Autodesk Inventor part; units mm, degrees
(part 3 of 3)
  arc A521 (160.6305, 133.2562) -> (159.9026, 133.5577) centre (148.5, 105) ccw projected
  arc A522 (159.9026, 133.5577) -> (159.9766, 134.127) centre (152.4268, 134.8199) ccw projected
  arc A523 (159.9766, 134.127) -> (160.0175, 134.9083) centre (150.1116, 135.0348) ccw projected
  arc A524 (160.0175, 134.9083) -> (159.988, 135.9358) centre (147.6733, 135.0675) ccw projected
  arc A525 (159.988, 135.9358) -> (159.2452, 136.2016) centre (148.5, 105) ccw projected
  arc A526 (159.2452, 136.2016) -> (158.5704, 135.426) centre (168.2137, 127.718) ccw projected
  arc A527 (158.5704, 135.426) -> (158.1064, 134.7962) centre (166.3081, 129.2396) ccw projected
  arc A528 (158.1064, 134.7962) -> (157.8025, 134.3091) centre (164.3821, 130.5422) ccw projected
  arc A529 (157.8025, 134.3091) -> (157.0485, 134.5379) centre (148.5, 105) ccw projected
  arc A530 (157.0485, 134.5379) -> (157.0664, 135.1116) centre (149.485, 135.0612) ccw projected
  arc A531 (157.0664, 135.1116) -> (157.0305, 135.8932) centre (147.1599, 135.0481) ccw projected
  arc A532 (157.0305, 135.8932) -> (156.9004, 136.9129) centre (144.7301, 134.8417) ccw projected
  arc A533 (156.9004, 136.9129) -> (156.1351, 137.1046) centre (148.5, 105) ccw projected
  arc A534 (156.1351, 137.1046) -> (155.5397, 136.2666) centre (165.892, 129.5409) ccw projected
  arc A535 (155.5397, 136.2666) -> (155.1396, 135.5943) centre (163.8464, 130.8684) ccw projected
  arc A536 (155.1396, 135.5943) -> (154.8849, 135.0798) centre (161.802, 131.976) ccw projected
  arc A537 (154.8849, 135.0798) -> (154.1121, 135.2335) centre (148.5, 105) ccw projected
  arc A538 (154.1121, 135.2335) -> (154.0737, 135.8063) centre (146.5338, 135.013) ccw projected
  arc A539 (154.0737, 135.8063) -> (153.9614, 136.5805) centre (144.2211, 134.7721) ccw projected
  arc A540 (153.9614, 136.5805) -> (153.7319, 137.5826) centre (141.8233, 134.3285) ccw projected
  arc A541 (153.7319, 137.5826) -> (152.9516, 137.6984) centre (148.5, 105) ccw projected
  arc A542 (152.9516, 137.6984) -> (152.4411, 136.8061) centre (163.4028, 131.1274) ccw projected
  arc A543 (152.4411, 136.8061) -> (152.1089, 136.0978) centre (161.237, 132.248) ccw projected
  arc A544 (152.1089, 136.0978) -> (151.9058, 135.5608) centre (159.0939, 133.1499) ccw projected
  arc A545 (151.9058, 135.5608) -> (151.1217, 135.638) centre (148.5, 105) ccw projected
  arc A546 (151.1217, 135.638) -> (151.0273, 136.2043) centre (143.6015, 134.6758) ccw projected
  arc A547 (151.0273, 136.2043) -> (150.8397, 136.9638) centre (141.3236, 134.2093) ccw projected
  arc A548 (150.8397, 136.9638) -> (150.5131, 137.9385) centre (138.9807, 133.5328) ccw projected
  arc A549 (150.5131, 137.9385) -> (149.7251, 137.9773) centre (148.5, 105) ccw projected
  arc A550 (149.7251, 137.9773) -> (149.3046, 137.0392) centre (160.7701, 132.4624) ccw projected
  arc A551 (149.3046, 137.0392) -> (149.0434, 136.3017) centre (158.5049, 133.3653) ccw projected
  point P0 (0, 0)
